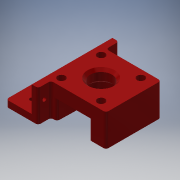
# Autodesk Inventor part: Y motor mount
Saved by Autodesk Inventor 2018 (Build 220112000, 112)
## iProperties
Part Number: Y motor mount
Material: ABS-Kunststoff
Document SubType Name: Modeling
Designer: Till
Density: 1.06 g/cm^3
Appearance: Rot
Author: Till
Autodesk Inventor part; units mm, degrees
ref_plane "YZ Plane" through (0, 0, 0) normal (1, 0, 0) x (0, 1, 0)
ref_plane "XZ Plane" through (0, 0, 0) normal (0, 1, 0) x (-1, 0, 0)
ref_plane "XY Plane" through (0, 0, 0) normal (0, 0, 1) x (1, 0, 0)
sketch "Skizze1" plane through (0, 0, 0) normal (0, 0, 1) x (1, 0, 0)
  line L0 (-22.6982, -31.5196) -> (-17.6982, -31.5196)
  line L1 (-17.6982, -31.5196) -> (-17.6982, -21.5196)
  line L2 (-17.6982, -21.5196) -> (25.3018, -21.5196)
  line L3 (25.3018, -21.5196) -> (25.3018, 21.4804)
  line L4 (25.3018, 21.4804) -> (-17.6982, 21.4804)
  line L5 (-17.6982, 21.4804) -> (-17.6982, 31.4804)
  line L6 (-17.6982, 31.4804) -> (-22.6982, 31.4804)
  line L7 (-22.6982, -31.5196) -> (-22.6982, 31.4804)
  point P0 (0, 0)
  dimension "d0" = 5
  dimension "d1" = 10
  dimension "d2" = 43
  dimension "d3" = 43
  dimension "d4" = 10
  dimension "d5" = 5
  constraints: 16 end point, 4 perpendicular, 2 point on line, 1 vertical
  measures "d0" distance of L0.start L0.end
  measures "d1" distance of L0.end L1.end
  measures "d2" distance of L1.end L2.end
  measures "d3" distance of L2.end L3.end
  measures "d4" distance of L4.end L5.end
  measures "d5" distance of L5.end L6.end
extrude "Extrusion1" add sketch "Skizze1" against normal blind 25
sketch "Skizze2" plane through (-22.6982, -31.5196, 0) normal (-1, 0, 0) x (0, 0, 1)
  line L0 (-25, 0) -> (-25, 63) projected
  line L1 (0, 63) -> (-25, 63) projected
  line L2 (-25, 0) -> (-20, 0)
  line L3 (-20, 0) -> (-20, 63)
  line L4 (-20, 63) -> (-25, 63)
  line L5 (-25, 63) -> (-25, 0)
  point P0 (0, 31.5196)
  dimension "d8" = 5
  constraints: 8 end point, 2 parallel, 1 horizontal, 1 perpendicular, 1 point on line
  measures "d8" distance of L4.end L3.end
extrude "Extrusion2" add sketch "Skizze2" along normal blind 20
sketch "Skizze3" plane through (0, 0, -25) normal (0, 0, -1) x (-1, 0, 0)
  line L0 (12.9973, -21.5196) -> (-12.0027, -21.5196)
  line L1 (12.9973, -21.5196) -> (12.4967, 0.2869)
  line L2 (-12.0027, -21.5196) -> (-12.4994, 0.1188)
  arc A0 (12.4967, 0.2869) -> (-12.4994, 0.1188) centre (0, 0) ccw
  dimension "d12" = 25
  constraints: 6 end point, 2 point on circle, 1 centre point, 1 coincident, 1 parallel
  measures "d12" distance of L0.start L0.end
extrude "Extrusion3" cut sketch "Skizze3" against normal blind 15
sketch "Skizze4" plane through (0, 0, -25) normal (0, 0, -1) x (-1, 0, 0)
  circle A0 centre (32.6982, -21.5196) radius 1.6
  line L0 (42.6982, 31.4804) -> (42.6982, -31.5196) projected
  line L1 (17.6982, -31.5196) -> (42.6982, -31.5196) projected
  circle A1 centre (32.6982, -1.5196) radius 1.6
  circle A2 centre (32.6982, 18.4804) radius 1.6
  point P0 (0, 0)
  dimension "d16" = 3.2
  dimension "d17" = 10
  dimension "d18" = 10
  dimension "d21" = 20
  constraints: 3 centre point, 1 vertical, 4 other
  measures "d16" diameter of A0
  measures "d17" distance from line of L0 A0.centre
  measures "d18" distance from line of L1 A0.centre
  measures "d21" distance of A0.centre A1.centre
extrude "Extrusion4" cut sketch "Skizze4" against normal through all
fillet "Rundung1" radius 2 10 edges at (25.3018, -21.5196, -12.5) (-17.6982, -21.5196, -12.5) (25.3018, 21.4804, -12.5) (-17.6982, 21.4804, -12.5) (-17.6982, 31.4804, -12.5) (-17.6982, -31.5196, -12.5) (-42.6982, -31.5196, -22.5) (-42.6982, 31.4804, -22.5) (-12.9973, -21.5196, -17.5) (12.0027, -21.5196, -17.5)
sketch "Skizze5" plane through (0, 0, -25) normal (0, 0, -1) x (-1, 0, 0)
  circle A0 centre (15.5, -15.5) radius 1.6
  circle A1 centre (-15.5, -15.5) radius 1.6
  circle A2 centre (15.5, 15.5) radius 1.6
  circle A3 centre (-15.5, 15.5) radius 1.6
  point P0 (0, 0)
  dimension "d29" = 3.2
  dimension "d30" = 15.5
  dimension "d31" = 15.5
  dimension "d32" = 3.2
  dimension "d33" = 31
  dimension "d34" = 3.2
  dimension "d35" = 3.2
  dimension "d36" = 31
  dimension "d37" = 31
  dimension "d38" = 31
  constraints: 4 centre point
  measures "d29" diameter of A0
  measures "d30" horizontal distance of point (0, 0) A0.centre
  measures "d31" horizontal distance of point (0, 0) A0.centre
  measures "d32" diameter of A1
  measures "d33" distance of A1.centre A0.centre
  measures "d34" diameter of A2
  measures "d35" diameter of A3
  measures "d36" distance of A2.centre A0.centre
  measures "d37" distance of A3.centre A2.centre
  measures "d38" distance of A1.centre A3.centre
extrude "Extrusion5" cut sketch "Skizze5" against normal through all
sketch "Skizze6" plane through (-17.6982, 23.4804, 0) normal (1, 0, 0) x (0, 0, -1)
  circle A0 centre (10, 3) radius 1.6
  line L0 (0, 0) -> (0, 6) projected
  line L1 (25, 8) -> (0, 8) projected
  circle A1 centre (10, -50) radius 1.6
  line L2 (0, -55) -> (25, -55) projected
  line L3 (0, -53) -> (0, -47) projected
  point P0 (0, -23.4804)
  dimension "d41" = 3.2
  dimension "d42" = 10
  dimension "d43" = 5
  dimension "d44" = 3.2
  dimension "d45" = 5
  dimension "d46" = 10
  constraints: 2 centre point
  measures "d41" diameter of A0
  measures "d42" distance from line of L0 A0.centre
  measures "d43" distance from line of L1 A0.centre
  measures "d44" diameter of A1
  measures "d45" distance from line of L2 A1.centre
  measures "d46" distance from line of L3 A1.centre
extrude "Extrusion6" cut sketch "Skizze6" against normal through all
sketch "Skizze7" plane through (0, 0, 0) normal (0, 0, 1) x (1, 0, 0)
  circle A0 centre (15.5, -15.5) radius 1.6 projected
  circle A1 centre (-15.5, -15.5) radius 1.6 projected
  circle A2 centre (-15.5, 15.5) radius 1.6 projected
  circle A3 centre (15.5, 15.5) radius 1.6 projected
  circle A4 centre (15.5, -15.5) radius 3
  circle A5 centre (-15.5, -15.5) radius 3
  circle A6 centre (15.5, 15.5) radius 1.6 projected
  circle A7 centre (15.5, 15.5) radius 3
  circle A8 centre (-15.5, 15.5) radius 3
  point P0 (0, 0)
  dimension "d49" = 6
  dimension "d50" = 6
  dimension "d51" = 6
  dimension "d52" = 6
  constraints: 4 centre point, 4 coincident
  measures "d49" diameter of A4
  measures "d50" diameter of A5
  measures "d51" diameter of A7
  measures "d52" diameter of A8
extrude "Extrusion7" cut sketch "Skizze7" against normal blind 8
sketch "Skizze8" plane through (0, 0, -10) normal (0, 0, -1) x (-1, 0, 0)
  circle A0 centre (0, 0) radius 8.5
  dimension "d55" = 17
  constraints: 1 centre point, 1 coincident
  measures "d55" diameter of A0
extrude "Extrusion8" cut sketch "Skizze8" against normal through all
chamfer "Fase1" distance 2 angle 45 2 edges at (8.5, 0, -10) (8.5, 0, 0)
